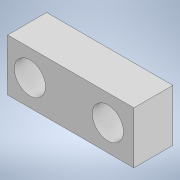
# Autodesk Inventor part: turntable_hit
Saved by Autodesk Inventor 2020 (Build 240168000, 168)
## iProperties
Created: 2020-10-21
Part Number: turntable_hit
Material: Generic
Document SubType Name: Modeling
Designer: s4393944
Density: 1 g/cm^3
Appearance: Default
Author: s4393944
Autodesk Inventor part; units mm, degrees
ref_plane "YZ Plane" through (0, 0, 0) normal (1, 0, 0) x (0, 1, 0)
ref_plane "XZ Plane" through (0, 0, 0) normal (0, 1, 0) x (-1, 0, 0)
ref_plane "XY Plane" through (0, 0, 0) normal (0, 0, 1) x (1, 0, 0)
sketch "Sketch1" plane through (0, 0, 0) normal (0, 0, 1) x (1, 0, 0)
  arc A0 (-243.5713, 10) -> (-243.5713, -10) centre (0, 0) ccw
  line L0 (-195, -10) -> (-195, 10)
  line L1 (-195, 10) -> (-243.5713, 10)
  line L2 (-195, -10) -> (-195, -10)
  line L3 (-195, -10) -> (-243.5713, -10)
  dimension "d19" = 10
  dimension "d20" = 10
  dimension "d21" = 0
  constraints: 8 end point, 2 point on circle, 1 centre point, 1 coincident, 1 horizontal, 1 perpendicular, 1 point on line
  measures "d19" vertical distance of L0.end point (0, 0)
  measures "d20" vertical distance of L2.end point (0, 0)
  measures "d21" vertical distance of L1.end L0.end
extrude "Extrusion1" add sketch "Sketch1" along normal blind 15
sketch "Sketch2" plane through (0, 0, 15) normal (0, 0, 1) x (1, 0, 0)
  circle A0 centre (-205, 0) radius 2.6
  line L0 (-195, -10) -> (-195, 10) projected
  circle A1 centre (-235, 0) radius 2.6
  point P0 (0, 0)
  dimension "d6" = 5.2
  dimension "d7" = 10
  dimension "d8" = 10
  dimension "d9" = 5.2
  dimension "d10" = 10
  dimension "d11" = 30
  constraints: 2 centre point
  measures "d6" diameter of A0
  measures "d7" distance from line of L0 A0.centre
  measures "d8" horizontal distance of L0.end A0.centre
  measures "d9" diameter of A1
  measures "d10" vertical distance of L0.end A1.centre
  measures "d11" distance of A0.centre A1.centre
hole "Hole1" at (-235, 0, 15) at (-205, 0, 15) direction (0, 0, -1) diameter 5.2 end through all counterbore diameter 12 counterbore depth 12
body "Solid1"
